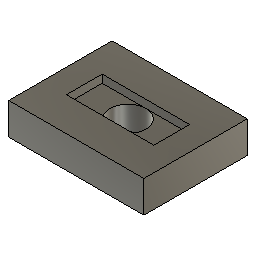
Base Block (Autodesk Fusion 360 design; units mm, degrees)
Autodesk Fusion 360 part; units mm, degrees
sketch "Sketch1" plane through (0, 0, 0) normal (0, 0, 1) x (1, 0, 0)
  circle A0 centre (0, 0) radius 4.5 construction
  line L0 (-11, 4.5) -> (11, 4.5) construction
  line L1 (11, 4.5) -> (11, -4.5) construction
  line L2 (11, -4.5) -> (-11, -4.5) construction
  line L3 (-11, -4.5) -> (-11, 4.5) construction
  line L4 (-17, 13) -> (17, 13)
  line L5 (17, 13) -> (17, -13)
  line L6 (17, -13) -> (-17, -13)
  line L7 (-17, -13) -> (-17, 13)
  dimension "d1" = 9
  dimension "d2" = 22
  dimension "d3" = 9
  dimension "d4" = 11
  dimension "d5" = 4.5
  dimension "d6" = 34
  dimension "d7" = 26
  dimension "d8" = 13
  dimension "d9" = 17
  constraint coincident A0.centre origin
  constraint horizontal L0
  constraint vertical L1
  constraint horizontal L2
  constraint vertical L3
  constraint horizontal L4
  constraint vertical L5
  constraint horizontal L6
  constraint vertical L7
  measures "d1" diameter of A0
  measures "d2" distance of L0.start L0.end
  measures "d3" distance of L0.start L2.end
  measures "d4" distance of A0.centre L3
  measures "d5" distance of A0.centre L0
  measures "d6" distance of L4.start L4.end
  measures "d7" distance of L4.start L6.end
  measures "d8" distance of A0.centre L4
  measures "d9" distance of A0.centre L5
extrude "Extrude1" add sketch "Sketch1" along normal blind 10
sketch "Sketch2" plane through (0, 0, 10) normal (0, 0, 1) x (-1, 0, 0)
  line L0 (17, 13) -> (-17, 13)
  line L1 (-17, 13) -> (-17, -13)
  line L2 (-17, -13) -> (17, -13)
  line L3 (17, -13) -> (17, 13)
  line L4 (11, -4.5) -> (-11, -4.5)
  line L5 (-11, -4.5) -> (-11, 4.5)
  line L6 (-11, 4.5) -> (11, 4.5)
  line L7 (11, 4.5) -> (11, -4.5)
  dimension "d12" = 22
  dimension "d13" = 9
  dimension "d14" = 11
  dimension "d15" = 4.5
  constraint horizontal L4
  constraint vertical L5
  constraint horizontal L6
  constraint vertical L7
  measures "d12" distance of L4.start L4.end
  measures "d13" distance of L4.start L6.end
  measures "d14" distance of origin L7
  measures "d15" distance of origin L4
extrude "Extrude2" cut sketch "Sketch2" against normal blind 2 contours L4 L5 L6 L7
extrude "Extrude3" cut 1 faces at (-5.6667, 4.3333, 0) along direction (0, 0, 1) blind 2
sketch "Sketch3" plane through (0, 0, 8) normal (0, 0, 1) x (-1, 0, 0)
  line L0 (11, 4.5) -> (-11, 4.5)
  line L1 (-11, 4.5) -> (-11, -4.5)
  line L2 (-11, -4.5) -> (11, -4.5)
  line L3 (11, -4.5) -> (11, 4.5)
  circle A0 centre (0, 0) radius 4.5
  dimension "d20" = 9
  constraint coincident A0.centre origin
  measures "d20" diameter of A0
extrude "Extrude4" cut sketch "Sketch3" against normal blind 26 contours A0
